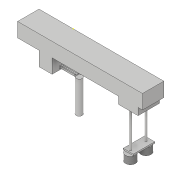
# Autodesk Inventor part: new part ee
Saved by Autodesk Inventor 2019 (Build 230136000, 136)
## iProperties
Created: 2019-11-24
Part Number: new part ee
Material: Generic
Document SubType Name: Sheet Metal
Designer: Mahesh
Density: 1 g/cm^3
Sheet Metal Rule: Default
Appearance: Default
Author: Mahesh
Autodesk Inventor part; units mm, degrees
ref_plane "YZ Plane" through (0, 0, 0) normal (1, 0, 0) x (0, 1, 0)
ref_plane "XZ Plane" through (0, 0, 0) normal (0, 1, 0) x (-1, 0, 0)
ref_plane "XY Plane" through (0, 0, 0) normal (0, 0, 1) x (1, 0, 0)
sketch "Sketch1" plane through (0, 0, 0) normal (0, 0, 1) x (1, 0, 0)
  line L0 (0, 0) -> (1750, 0)
  line L1 (1750, 0) -> (1750, -200)
  line L2 (1750, -200) -> (0, -200)
  line L3 (0, -200) -> (0, 0)
  dimension "d0" = 1750
  dimension "d1" = 200
  constraints: 8 end point, 2 parallel, 1 horizontal, 1 perpendicular
  measures "d0" distance of L1.end L2.end
  measures "d1" distance of L0.end L1.end
extrude "Extrusion1" add sketch "Sketch1" along normal blind 300
sketch "Sketch2" plane through (0, -200, 0) normal (0, -1, 0) x (1, 0, 0)
  line L0 (1750, 300) -> (0, 300) projected
  line L1 (146.9442, 300) -> (146.9442, 150.1387)
  circle A0 centre (146.9442, 150.1387) radius 66.1557
  point P0 (0, 0)
  constraints: 2 end point, 1 centre point, 1 coincident, 1 point on line, 1 vertical
extrude "Extrusion2" add sketch "Sketch2" against normal blind 150
sketch "Sketch3" plane through (0, -200, 0) normal (0, -1, 0) x (1, 0, 0)
  line L0 (1750, 300) -> (0, 300) projected
  line L1 (146.9442, 300) -> (146.9442, 150.1387)
  circle A0 centre (146.9442, 150.1387) radius 47.6199
  point P0 (0, 0)
  constraints: 2 end point, 1 centre point, 1 coincident, 1 point on line, 1 vertical
extrude "Extrusion3" cut sketch "Sketch3" against normal blind 150
sketch "Sketch4" plane through (0, -200, 0) normal (0, -1, 0) x (1, 0, 0)
  line L0 (0, 300) -> (1750, 300) projected
  line L1 (1750, 0) -> (0, 0) projected
  line L2 (300.2774, 300) -> (483.4253, 300)
  line L3 (483.4253, 300) -> (483.4253, 0)
  line L4 (483.4253, 0) -> (300.2774, 0)
  line L5 (300.2774, 0) -> (300.2774, 300)
  constraints: 8 end point, 2 parallel, 2 point on line, 1 horizontal, 1 perpendicular
extrude "Extrusion4" add sketch "Sketch4" along normal blind 200
sketch "Sketch5" plane through (483.4253, -200, 300) normal (1, 0, 0) x (0, 0, -1)
  point P0 (300, 200)
sketch "Sketch6" plane through (483.4253, -200, 300) normal (1, 0, 0) x (0, 0, -1)
  line L0 (104.45, -150.7604) -> (197.7293, -150.7604)
  line L1 (197.7293, -150.7604) -> (197.7293, -187.6383)
  line L2 (197.7293, -187.6383) -> (104.45, -187.6383)
  line L3 (104.45, -187.6383) -> (104.45, -150.7604)
  point P0 (300, 200)
  constraints: 8 end point, 2 parallel, 1 horizontal, 1 perpendicular
extrude "Extrusion5" cut sketch "Sketch6" against normal blind 170
sketch "Sketch7" plane through (483.4253, -200, 300) normal (1, 0, 0) x (0, 0, -1)
  line L0 (197.7293, -187.6383) -> (104.45, -187.6383) projected
  line L1 (119.9492, -187.6383) -> (180.6892, -187.6383)
  line L2 (180.6892, -187.6383) -> (180.6892, -163.3555)
  line L3 (180.6892, -163.3555) -> (119.9492, -163.3555)
  line L4 (119.9492, -163.3555) -> (119.9492, -187.6383)
  point P0 (300, 200)
  constraints: 8 end point, 2 parallel, 1 horizontal, 1 perpendicular, 1 point on line
extrude "Extrusion6" add sketch "Sketch7" along normal blind 200
sketch "Sketch8" plane through (683.4253, -200, 300) normal (1, 0, 0) x (0, 0, -1)
  line L0 (180.6892, -163.3555) -> (119.9492, -163.3555) projected
  line L1 (132.9649, -163.3555) -> (163.3349, -163.3555)
  line L2 (163.3349, -163.3555) -> (163.3349, -176.3712)
  line L3 (163.3349, -176.3712) -> (132.9649, -176.3712)
  line L4 (132.9649, -176.3712) -> (132.9649, -163.3555)
  point P0 (300, 200)
  constraints: 8 end point, 2 parallel, 1 horizontal, 1 perpendicular, 1 point on line
extrude "Extrusion7" cut sketch "Sketch8" against normal blind 200
sketch "Sketch9" plane through (483.4253, -387.6383, 119.3108) normal (0, -1, 0) x (1, 0, 0)
  circle A0 centre (232.1912, 32.9184) radius 42.3537
  point P0 (-483.4253, -119.3108)
  constraints: 1 centre point
extrude "Extrusion8" add sketch "Sketch9" along normal blind 450
sketch "Sketch10" plane through (715.6165, -837.6383, 152.2291) normal (0, -1, 0) x (1, 0, 0)
  circle A0 centre (0, 0) radius 27.7499
  point P0 (-715.6165, -152.2291)
  constraints: 1 centre point
extrude "Extrusion9" cut sketch "Sketch10" against normal blind 250
sketch "Sketch11" plane through (1750, -200, 0) normal (0, -1, 0) x (1, 0, 0)
  line L0 (-1266.5747, 300) -> (0, 300) projected
  line L1 (-333.395, 300) -> (-61.3169, 300)
  line L2 (-61.3169, 300) -> (-61.3169, 0)
  line L3 (-61.3169, 0) -> (-333.395, 0)
  line L4 (-333.395, 0) -> (-333.395, 300)
  point P0 (-1750, 0)
  constraints: 8 end point, 2 parallel, 1 horizontal, 1 perpendicular, 1 point on line
extrude "Extrusion10" add sketch "Sketch11" along normal blind 100
sketch "Sketch12" plane through (1750, -300, 0) normal (0, -1, 0) x (1, 0, 0)
  line L0 (0, 300) -> (-1750, 300) projected
  line L1 (-198.623, 300) -> (-198.623, 250.4175)
  line L2 (-1750, 0) -> (0, 0) projected
  line L3 (-198.623, 0) -> (-198.623, 51.3474)
  circle A0 centre (-198.623, 250.4175) radius 12.6394
  circle A1 centre (-198.623, 51.3474) radius 12.6394
  constraints: 4 end point, 2 centre point, 2 coincident, 2 point on line, 1 perpendicular, 1 vertical
extrude "Extrusion11" add sketch "Sketch12" along normal blind 500 contours A1
sketch "Sketch13" plane through (1750, -300, 0) normal (0, -1, 0) x (1, 0, 0)
  circle A0 centre (-197.356, 270.3298) radius 13.7095
  point P0 (-1750, 0)
  constraints: 1 centre point
extrude "Extrusion12" add sketch "Sketch13" along normal blind 500
sketch "Sketch14" plane through (1552.644, -800, 270.3298) normal (0, -1, 0) x (1, 0, 0)
  line L0 (197.356, 29.6702) -> (-1552.644, 29.6702) projected
  line L1 (-1552.644, -270.3298) -> (197.356, -270.3298) projected
  line L2 (68.9898, 29.6702) -> (-72.1361, 29.6702)
  line L3 (-72.1361, 29.6702) -> (-72.1361, -270.3298)
  line L4 (-72.1361, -270.3298) -> (68.9898, -270.3298)
  line L5 (68.9898, -270.3298) -> (68.9898, 29.6702)
  constraints: 8 end point, 2 parallel, 2 point on line, 1 horizontal, 1 perpendicular
extrude "Extrusion13" add sketch "Sketch14" along normal blind 20
sketch "Sketch15" plane through (1552.644, -820, 270.3298) normal (0, -1, 0) x (1, 0, 0)
  circle A0 centre (0, 0) radius 13.7095 projected
  circle A1 centre (0, 0) radius 13.7095
  circle A2 centre (-1.2671, -218.9824) radius 12.6394 projected
  circle A3 centre (-1.2671, -218.9824) radius 12.6394
  point P0 (-1552.644, -270.3298)
  constraints: 2 centre point, 2 coincident
extrude "Extrusion14" add sketch "Sketch15" along normal blind 10 contours A2
sketch "Sketch16" plane through (1552.644, -820, 270.3298) normal (0, -1, 0) x (1, 0, 0)
  circle A0 centre (0, 0) radius 13.7095 projected
  circle A1 centre (0, 0) radius 13.7095
  point P0 (-1552.644, -270.3298)
  constraints: 1 centre point, 1 coincident
extrude "Extrusion15" add sketch "Sketch16" along normal blind 10
sketch "Sketch17" plane through (1552.644, -830, 270.3298) normal (0, -1, 0) x (1, 0, 0)
  circle A0 centre (0, 0) radius 13.7095 projected
  circle A1 centre (0, 0) radius 68.9898
  line L0 (68.9898, -270.3298) -> (68.9898, 29.6702) projected
  circle A2 centre (-1.2671, -218.9824) radius 12.6394 projected
  circle A3 centre (-1.2671, -218.9824) radius 70.2568
  point P0 (-1552.644, -270.3298)
  constraints: 2 centre point, 2 coincident, 2 tangent
extrude "Extrusion16" add sketch "Sketch17" along normal blind 100 contours A1
sketch "Sketch18" plane through (1551.377, -830, 51.3474) normal (0, -1, 0) x (1, 0, 0)
  circle A0 centre (0, 0) radius 12.6394 projected
  circle A1 centre (0, 0) radius 70.2568
  line L0 (70.2568, -51.3474) -> (70.2568, 248.6526) projected
  point P0 (-1551.377, -51.3474)
  constraints: 1 centre point, 1 coincident, 1 tangent
extrude "Extrusion17" add sketch "Sketch18" along normal blind 100
thread "Thread1" size "M140x8" class "6g" standard "ANSI Metric M Profile" full length
thread "Thread2" size "M145x6" class "6g" standard "ANSI Metric M Profile" full length
thread "Thread3" size "M56x6.5" class "6H" standard "ANSI Metric M Profile" full length
equation "\"BendRadius\" = Thickness"
equation "\"BendReliefWidth\" = Thickness"
equation "\"BendReliefDepth\" = 0.5 * Thickness"
equation "\"CornerReliefSize\" = 4 * Thickness"
equation "\"MinimumRemnant\" = 2 * Thickness"
equation "\"TransitionRadius\" = BendRadius"
equation "\"JacobiRadiusSize\" = BendRadius"
equation "\"GapSize\" = Thickness"
equation "\"Thickness\" = 3.048"
body "Solid1"
